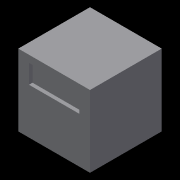
# Autodesk Inventor part: open reflow box
Saved by Autodesk Inventor 2013 (Build 170138000, 138)
## iProperties
Created: 2012-12-28
Part Number: open reflow box
Material: Generic
Document SubType Name: Modeling
Designer: Administrator
Density: 1 g/cm^3
Author: Administrator
Autodesk Inventor part; units mm, degrees
ref_plane "YZ Plane" through (0, 0, 0) normal (1, 0, 0) x (0, 1, 0)
ref_plane "XZ Plane" through (0, 0, 0) normal (0, 1, 0) x (-1, 0, 0)
ref_plane "XY Plane" through (0, 0, 0) normal (0, 0, 1) x (1, 0, 0)
sketch "Sketch1" plane through (0, 0, 0) normal (0, 0, 1) x (1, 0, 0)
  line L0 (-51.5546, 67.657) -> (50.0454, 67.657)
  line L1 (50.0454, 67.657) -> (50.0454, -33.943)
  line L2 (50.0454, -33.943) -> (-51.5546, -33.943)
  line L3 (-51.5546, -33.943) -> (-51.5546, 67.657)
  line L4 (-25.4, 55.5625) -> (15.875, 55.5625)
  line L5 (15.875, 55.5625) -> (15.875, -15.0495)
  line L6 (15.875, -15.0495) -> (-25.4, -15.0495)
  line L7 (-25.4, -15.0495) -> (-25.4, 55.5625)
  line L8 (-21.8726, 53.0629) -> (11.8332, 53.0629)
  line L9 (11.8332, 53.0629) -> (11.8332, 24.8943)
  line L10 (11.8332, 24.8943) -> (-21.8726, 24.8943)
  line L11 (-21.8726, 24.8943) -> (-21.8726, 53.0629)
  line L12 (12.194, -13.9931) -> (-21.5118, -13.9931)
  line L13 (-21.5118, -13.9931) -> (-21.5118, 14.1755)
  line L14 (-21.5118, 14.1755) -> (12.194, 14.1755)
  line L15 (12.194, 14.1755) -> (12.194, -13.9931)
  point P0 (0, 0)
  dimension "d0" = 101.6
  dimension "d2" = 101.6
  dimension "d35" = 41.275
  dimension "d36" = 70.612
  dimension "d37" = 33.7058
  dimension "d38" = 28.1686
  dimension "d39" = 33.7058
  dimension "d40" = 28.1686
  constraints: 32 end point, 8 parallel, 4 horizontal, 4 perpendicular
  measures "d0" distance of L2.end L0.start
  measures "d2" distance of L0.start L0.end
  measures "d35" distance of L4.start L4.end
  measures "d36" distance of L4.end L5.end
  measures "d37" distance of L8.start L8.end
  measures "d38" distance of L10.end L8.start
  measures "d39" distance of L13.end L14.end
  measures "d40" distance of L12.end L13.end
extrude "Extrusion1" add sketch "Sketch1" against normal blind 101.6 contours L0 L1 L2 L3 | L4 L5 L6 L7 | L8 L9 L10 L11 | L12 L13 L14 L15
sketch "Sketch2" plane through (0, 0, 0) normal (0, 0, 1) x (1, 0, 0)
  circle A0 centre (-38.7804, 61.0277) radius 1.25
  circle A1 centre (-38.7804, 30.0277) radius 1.25
  circle A2 centre (36.2196, 61.0277) radius 1.25
  circle A3 centre (36.2196, 30.0277) radius 1.25
  line L0 (-36.3665, 57.6923) -> (34.9335, 57.6923)
  line L1 (34.9335, 57.6923) -> (34.9335, 30.8923)
  line L2 (34.9335, 30.8923) -> (-36.3665, 30.8923)
  line L3 (-36.3665, 30.8923) -> (-36.3665, 57.6923)
  line L4 (34.9013, 51.3389) -> (37.4013, 51.3389)
  line L5 (37.4013, 51.3389) -> (37.4013, 37.5389)
  line L6 (37.4013, 37.5389) -> (34.9013, 37.5389)
  line L7 (34.9013, 37.5389) -> (34.9013, 51.3389)
  line L8 (-38.8519, 51.3389) -> (-36.3519, 51.3389)
  line L9 (-36.3519, 51.3389) -> (-36.3519, 37.5389)
  line L10 (-36.3519, 37.5389) -> (-38.8519, 37.5389)
  line L11 (-38.8519, 37.5389) -> (-38.8519, 51.3389)
  point P0 (0, 0)
  constraints: 24 end point, 6 parallel, 4 centre point, 3 horizontal, 3 perpendicular
extrude "Extrusion2" cut sketch "Sketch2" against normal blind 5 contours L0 L1 L4 L7 L6 L2 L3 L10 L9 L8 | L8 L9 L10 L3 | L1 L6 L7 L4
body "Solid1"
